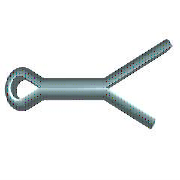
# Autodesk Inventor part: 100003
Saved by Autodesk Inventor 2020.1 (Build 241239000, 239)
## iProperties
Created: 2006-01-26
Part Number: 100003
Material: Steel, Mild
Description: Split Pin
Document SubType Name: Modeling
Standard: ISO 1234
Designer: Kevin
Standard Revision: Second edition 1997-11-01
Standards Organization: ISO
Language: en-US
Size Designation: 2.5 x 20
Categories: <MemberInstance><Categories><Category DisplayName="Fasteners" InternalName="e4da775c-781d-43d5-af7c-5136215cf5a6" Mnemonic="FSTN"><Category DisplayName="Pins" InternalName="3b3d1810-ac9b-4ede-8c7f-cc6b956350b0" Mnemonic="PIN"><CategoryParameter DisplayName="Nominal Diameter" InternalName="6cc331d7-8ea1-4fca-9c9a-55ec966217e5" Mnemonic="nomdia"/><CategoryParameter DisplayName="Nominal Length" InternalName="897bd938-6adf-4e3c-a2d4-0d7cae45eecd" Mnemonic="nomlen"/><Category DisplayName="Cotter Pins" InternalName="4383ab9c-662d-4701-a95a-d5834a9f0a34" Mnemonic="SPLTPIN"><CategoryParameter DisplayName="Bolt Diameter" InternalName="761c08f3-f58b-48c9-8a5c-1931069602db" Mnemonic="bltdia"/></Category></Category></Category></Categories><FamilyTemplate Id="si0028"><FamilyTemplateParameters><FamilyTemplateParameter ObjectType="kUserParameterObject" ValueType="xs:double" Id="1" ObjectReferenceKey="KBR"/><FamilyTemplateParameter ObjectType="kUserParameterObject" ValueType="xs:double" Id="2" ObjectReferenceKey="NNDMAX"/><FamilyTemplateParameter ObjectType="kUserParameterObject" ValueType="xs:double" Id="3" ObjectReferenceKey="DSH"/><FamilyTemplateParameter ObjectType="kUserParameterObject" ValueType="xs:double" Id="4" ObjectReferenceKey="MSIAB"/><FamilyTemplateParameter ObjectType="kUserParameterObject" ValueType="xs:double" Id="5" ObjectReferenceKey="SNLG"/><FamilyTemplateParameter ObjectType="kUserParameterObject" ValueType="xs:double" Id="6" ObjectReferenceKey="SNND"/><FamilyTemplateParameter ObjectType="kUserParameterObject" ValueType="xs:double" Id="7" ObjectReferenceKey="KOL"/><FamilyTemplateParameter ObjectType="kUserParameterObject" ValueType="xs:double" Id="8" ObjectReferenceKey="LGDIF"/><FamilyTemplateParameter ObjectType="kUserParameterObject" ValueType="xs:double" Id="9" ObjectReferenceKey="NNDMIN"/><FamilyTemplateParameter ObjectType="kUserParameterObject" ValueType="xs:double" Id="10" ObjectReferenceKey="SNND1"/><FamilyTemplateParameter ObjectType="kPropertyObject" ValueType="xs:string" Id="100" ObjectReferenceKey="{32853F0F-3444-11D1-9E93-0060B03C1CA6}" SubObjectId="52"/><FamilyTemplateParameter ObjectType="kPropertyObject" ValueType="xs:string" Id="101" ObjectReferenceKey="{32853F0F-3444-11D1-9E93-0060B03C1CA6}" SubObjectId="49"/><FamilyTemplateParameter ObjectType="kPropertyObject" ValueType="xs:string" Id="102" ObjectReferenceKey="{32853F0F-3444-11D1-9E93-0060B03C1CA6}" SubObjectId="37"/><FamilyTemplateParameter ObjectType="kPropertyObject" ValueType="xs:string" Id="103" ObjectReferenceKey="{32853F0F-3444-11D1-9E93-0060B03C1CA6}" SubObjectId="47"/><FamilyTemplateParameter ObjectType="kPropertyObject" ValueType="xs:string" Id="104" ObjectReferenceKey="{32853F0F-3444-11D1-9E93-0060B03C1CA6}" SubObjectId="48"/><FamilyTemplateParameter ObjectType="kPropertyObject" ValueType="xs:string" Id="105" ObjectReferenceKey="{32853F0F-3444-11D1-9E93-0060B03C1CA6}" SubObjectId="5"/><FamilyTemplateParameter ObjectType="kPropertyObject" ValueType="xs:string" Id="106" ObjectReferenceKey="{32853F0F-3444-11D1-9E93-0060B03C1CA6}" SubObjectId="29"/><FamilyTemplateParameter ObjectType="kPropertyObject" ValueType="xs:string" Id="107" ObjectReferenceKey="{32853F0F-3444-11D1-9E93-0060B03C1CA6}" SubObjectId="20"/><FamilyTemplateParameter ObjectType="kPropertyObject" ValueType="xs:string" Id="108" ObjectReferenceKey="{B9600981-DEE8-4547-8D7C-E525B3A1727A}" SubObjectId="17"/><FamilyTemplateParameter ObjectType="kPropertyObject" ValueType="xs:string" Id="109" ObjectReferenceKey="{B9600981-DEE8-4547-8D7C-E525B3A1727A}" SubObjectId="19"/><FamilyTemplateParameter ObjectType="kPropertyObject" ValueType="xs:string" Id="110" ObjectReferenceKey="{B9600981-DEE8-4547-8D7C-E525B3A1727A}" SubObjectId="21"/><FamilyTemplateParameter ObjectType="kPropertyObject" ValueType="xs:string" Id="111" ObjectReferenceKey="{B9600981-DEE8-4547-8D7C-E525B3A1727A}" SubObjectId="9"/><FamilyTemplateParameter ObjectType="kPartDocumentObject" ValueType="xs:string" Id="112" ObjectReferenceKey="" SubObjectId="DisplayName"/><FamilyTemplateParameter ObjectType="kPartFeatureObject" ValueType="xs:string" Id="400" ObjectReferenceKey="100200001000000039030000000000008000000000000000" SubObjectId="Name"/><FamilyTemplateParameter ObjectType="kPartFeatureObject" ValueType="xs:string" Id="401" ObjectReferenceKey="1002000010000000fb040000000000008000000000000000" SubObjectId="Name"/><FamilyTemplateParameter ObjectType="kPartFeatureObject" ValueType="xs:string" Id="402" ObjectReferenceKey="100200001000000086000000000000008000000000000000" SubObjectId="Name"/><FamilyTemplateParameter ObjectType="kiMateDefinitionObject" ValueType="xs:string" Id="500" ObjectReferenceKey="04010100100000000b43b64d19432353a33b8aa982ea62cf" SubObjectId="Name"/><FamilyTemplateParameter ObjectType="kiMateDefinitionObject" ValueType="xs:string" Id="501" ObjectReferenceKey="040101001000000034e9d25a864ebb901d0c0bacdf7e984a" SubObjectId="Name"/><FamilyTemplateParameter ObjectType="kiMateDefinitionObject" ValueType="xs:string" Id="502" ObjectReferenceKey="0401010010000000879ad30ca74bd793ea8f6e916b8451f6" SubObjectId="Name"/><FamilyTemplateParameter ObjectType="kiMateDefinitionObject" ValueType="xs:string" Id="503" ObjectReferenceKey="0401010010000000dd4a8713fd49d1a979ad11b5f1955a6f" SubObjectId="Name"/><FamilyTemplateParameter ObjectType="kiPartTableColumnObject" ValueType="xs:string" Id="504" ObjectReferenceKey="RID"/></FamilyTemplateParameters></FamilyTemplate><CategoryParameterMap><ParamToTemplateMap><ParamToTemplate CategoryParameter="//CategoryParameter[@InternalName='2675968c-4ce5-49e0-a4f5-552d29089031']" TemplateParameter="100"/><ParamToTemplate CategoryParameter="//CategoryParameter[@InternalName='8b46a4cc-9585-4fed-90c3-899f57e09a73']" TemplateParameter="110"/><ParamToTemplate CategoryParameter="//CategoryParameter[@InternalName='818a152a-d3c3-49ca-80ee-df7d91421b8e']" TemplateParameter="107"/><ParamToTemplate CategoryParameter="//CategoryParameter[@InternalName='761c08f3-f58b-48c9-8a5c-1931069602db']" TemplateParameter="2"/><ParamToTemplate CategoryParameter="//CategoryParameter[@InternalName='016b6077-bfbe-49bd-92c9-d8d59c39c941']" TemplateParameter="105"/><ParamToTemplate CategoryParameter="//CategoryParameter[@InternalName='8e5e0294-fc51-4c8f-b3d7-003dc5ed94f6']" TemplateParameter="504"/><ParamToTemplate CategoryParameter="//CategoryParameter[@InternalName='897bd938-6adf-4e3c-a2d4-0d7cae45eecd']" TemplateParameter="5"/><ParamToTemplate CategoryParameter="//CategoryParameter[@InternalName='6cc331d7-8ea1-4fca-9c9a-55ec966217e5']" TemplateParameter="6"/></ParamToTemplateMap></CategoryParameterMap></MemberInstance>
Density: 7.85 g/cm^3
Appearance: Steel
Mass: 0.998194 g
Volume: 0.127159 cm^3
Author: Kevin
Autodesk Inventor part; units mm, degrees
ref_plane "YZ Plane" through (0, 0, 0) normal (1, 0, 0) x (0, 1, 0)
sketch "Sketch1" plane through (0, 0, 0) normal (0, 1, 0) x (-1, 0, 0)
  arc A0 (-1.6014, 2.0207) -> (-1.6014, -2.0207) centre (-2.7, 0) ccw
  arc A1 (-2.2102, 1.0405) -> (-2.2102, -1.0405) centre (-2.7, 0) ccw
  line L0 (0, 1.15) -> (14, 1.15)
  line L1 (0, -1.15) -> (14, -1.15)
  line L2 (14, 1.15) -> (20, 3.4487)
  line L3 (20, 3.4487) -> (20.3842, 2.4459)
  line L4 (20.3842, 2.4459) -> (14, 0)
  line L5 (14, 0) -> (22.8842, -3.4037)
  line L6 (22.8842, -3.4037) -> (22.5, -4.4065)
  line L7 (22.5, -4.4065) -> (14, -1.15)
  line L8 (0, 0) -> (-2.2102, -1.0405)
  line L9 (0, 0) -> (-2.2102, 1.0405)
  line L10 (0, 1.15) -> (0, -1.15) construction
  line L11 (0, 1.15) -> (-1.6014, 2.0207)
  line L12 (0, -1.15) -> (-1.6014, -2.0207)
  line L13 (-5, 0) -> (14, 0) construction
  line L14 (14, 1.15) -> (14, -1.15) construction
  dimension "d0" = 14
  dimension "d1" = 20
  dimension "d2" = 159.037
  dimension "d3" = 159.037
  dimension "d4" = 2.5
  dimension "d5" = 1.15
  dimension "d6" = 2.3
  dimension "d7" = 1.15
  dimension "d8" = 1.15
  dimension "d9" = 2.7
  constraints: 30 end point, 5 point on circle, 4 parallel, 4 perpendicular, 4 point on line, 4 tangent, 2 centre point, 2 midpoint, 1 coincident, 1 horizontal
  measures "d0" distance of L0.start L0.end
  measures "d1" horizontal distance of L0.start L2.end
  measures "d2" angle of L0 L2
  measures "d3" angle of L1 L7
  measures "d4" horizontal distance of L2.end L6.end
  measures "d5" radius of A1
  measures "d6" radius of A0
  measures "d7" distance from line of L0 L8.start
  measures "d8" distance between parallel lines of L1 L13
  measures "d9" distance from line of L10 A0.centre
extrude "Body" add sketch "Sketch1" along normal mid plane 2.3
fillet "Fillet" radius 0.805 14 edges at (-17, -1.15, 2.2994) (-17, 1.15, 2.2994) (-7, -1.15, 1.15) (-7, 1.15, 1.15) (5, -1.15, 0) (0.8007, -1.15, -1.5853) (0.8007, -1.15, 1.5853) (5, 1.15, 0) (0.8007, 1.15, 1.5853) (0.8007, 1.15, -1.5853) (-7, -1.15, -1.15) (-18.25, -1.15, -2.7783) (-7, 1.15, -1.15) (-18.25, 1.15, -2.7783)
ref_plane "Work Plane1" through (0, -10, 0) normal (0, 0, -1) x (0, 1, 0)
ref_plane "Work Plane3" through (0, 0, 1.15) normal (-1, 0, 0) x (0, 1, 0)
equation "\"d0\" = MSIAB"
equation "\"d1\" = SNLG"
equation "\"d4\" = LGDIF"
equation "\"d5\" = -0.5 * SNND1 + 0.5 * KBR"
equation "\"d6\" = 0.5 * KBR"
equation "\"d7\" = 0.5 * SNND1"
equation "\"d8\" = 0.5 * SNND1"
equation "\"d9\" = KOL - 0.5 * KBR"
equation "\"d10\" = SNND1"
equation "\"d12\" = 0.35 * SNND1"
equation "\"SNND\" = 2.5"
equation "\"SNLG\" = 20"
equation "\"SNND1\" = 2.3"
equation "\"KBR\" = 4.6"
equation "\"KOL\" = 5"
equation "\"LGDIF\" = 2.5"
equation "\"MSIAB\" = 14"
equation "\"NNDMAX\" = 11"
equation "\"DSH\" = 5"
equation "\"NNDMIN\" = 9"
body "Solid1"
